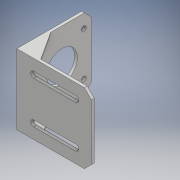
# Autodesk Inventor part: mount-extruder
Saved by Autodesk Inventor 2018 (Build 220112000, 112)
## iProperties
Created: 2017-10-21
Part Number: mount-extruder
Material: Generic
Document SubType Name: Modeling
Designer: Jurjen
Density: 1 g/cm^3
Appearance: Default
Author: Jurjen
Autodesk Inventor part; units mm, degrees
ref_plane "YZ Plane" through (0, 0, 0) normal (1, 0, 0) x (0, 1, 0)
ref_plane "XZ Plane" through (0, 0, 0) normal (0, 1, 0) x (-1, 0, 0)
ref_plane "XY Plane" through (0, 0, 0) normal (0, 0, 1) x (1, 0, 0)
sketch "Sketch1" plane through (0, 0, 0) normal (0, 0, 1) x (1, 0, 0)
  line L0 (-26.5, 25.5) -> (-24.5, 25.5)
  line L1 (-24.5, 25.5) -> (-24.5, -23.5)
  line L2 (-26.5, -25.5) -> (26.5, -25.5)
  line L3 (26.5, -25.5) -> (26.5, -23.5)
  line L4 (26.5, -23.5) -> (-24.5, -23.5)
  line L5 (-26.5, 25.5) -> (-26.5, -25.5)
  point P0 (0, 0)
  point P1 (-26.5, 0)
  point P2 (0, -25.5)
  dimension "d1" = 51
  dimension "d2" = 2
  dimension "d4" = 2
  dimension "d5" = 53
  constraints: 12 end point, 2 horizontal, 2 midpoint, 2 parallel, 2 perpendicular, 1 horizontal alignment, 1 vertical alignment
  measures "d1" distance of L0.start L2.start
  measures "d2" distance between parallel lines of L2 L4
  measures "d4" distance between parallel lines of L1 L5
  measures "d5" distance between parallel lines of L3 L5
extrude "Extrusion1" add sketch "Sketch1" along normal mid plane 50
sketch "Sketch2" plane through (-24.5, -23.5, 25) normal (1, 0, 0) x (0, 0, -1)
  circle A0 centre (25, 28) radius 11.05
  circle A1 centre (9.5, 43.5) radius 1.75
  circle A2 centre (40.5, 43.5) radius 1.75
  circle A3 centre (9.5, 12.5) radius 1.75
  circle A4 centre (40.5, 12.5) radius 1.75
  line L0 (0, 49) -> (50, 49) projected
  line L1 (9.5, 43.5) -> (40.5, 43.5) construction
  line L2 (9.5, 43.5) -> (9.5, 12.5) construction
  point P0 (25, 23.5)
  point P1 (25, 43.5)
  point P2 (9.5, 28)
  dimension "d8" = 22.1
  dimension "d9" = 3.5
  dimension "d10" = 31
  dimension "d11" = 31
  dimension "d12" = 21
  constraints: 5 centre point, 4 end point, 4 vertical alignment, 3 equal radius, 3 horizontal alignment, 2 midpoint, 1 horizontal, 1 vertical
  measures "d8" diameter of A0
  measures "d9" diameter of A1
  measures "d10" distance of L1.end L1.start
  measures "d11" distance of A4.centre L1.end
  measures "d12" distance from line of A0.centre L0
extrude "Extrusion2" cut sketch "Sketch2" against normal up to next
sketch "Sketch3" plane through (-24.5, -23.5, 25) normal (1, 0, 0) x (0, 0, -1)
  line L0 (0, 44) -> (5, 49)
  line L1 (50, 49) -> (0, 49) projected
  line L2 (25, 22.7162) -> (25, 49) construction
  line L3 (50, 44) -> (45, 49)
  line L4 (0, 0) -> (0, 49) projected
  line L5 (50, 49) -> (50, 0) projected
  line L6 (0, 49) -> (50, 49) projected
  line L7 (45, 49) -> (50, 49)
  line L8 (50, 49) -> (50, 44)
  line L9 (5, 49) -> (0, 49)
  line L10 (0, 44) -> (0, 49)
  point P0 (25, 23.5)
  dimension "d15" = 45
  dimension "d16" = 5
  constraints: 14 end point, 3 collinear, 2 symmetric about line, 2 vertical alignment, 1 midpoint, 1 perpendicular, 1 point on line
  measures "d15" angle of L1 L0
  measures "d16" distance of L1.end L0.end
extrude "Extrusion3" cut sketch "Sketch3" against normal up to next
sketch "Sketch4" plane through (-24.5, -23.5, 25) normal (0, 1, 0) x (1, 0, 0)
  arc A0 (10, 12.1) -> (10, 7.9) centre (10, 10) ccw
  arc A1 (10, 42.1) -> (10, 37.9) centre (10, 40) ccw
  arc A2 (40, 7.9) -> (40, 12.1) centre (40, 10) ccw
  arc A3 (40, 37.9) -> (40, 42.1) centre (40, 40) ccw
  line L0 (40, 7.9) -> (10, 7.9)
  line L1 (10, 12.1) -> (40, 12.1)
  line L2 (10, 37.9) -> (40, 37.9)
  line L3 (10, 42.1) -> (40, 42.1)
  line L4 (10, 10) -> (10, 40) construction
  line L5 (51, 50) -> (51, 0) projected
  point P0 (24.5, 25)
  point P1 (10, 25)
  dimension "d19" = 4.2
  dimension "d20" = 30
  dimension "d21" = 30
  dimension "d22" = 4.2
  dimension "d23" = 11
  constraints: 10 end point, 8 point on circle, 4 centre point, 3 equal radius, 3 horizontal alignment, 3 parallel, 3 tangent, 2 vertical alignment, 1 horizontal, 1 midpoint, 1 vertical
  measures "d19" diameter of A0
  measures "d20" distance of L4.start L4.end
  measures "d21" distance of L4.start A2.centre
  measures "d22" distance between parallel lines of L3 L2
  measures "d23" distance from line of L5 A3.centre
extrude "Extrusion4" cut sketch "Sketch4" against normal up to next
sketch "Sketch5" plane through (-24.5, -23.5, 25) normal (0, 1, 0) x (1, 0, 0)
  line L0 (10, 12.1) -> (40, 12.1) projected
  arc A0 (40, 7.9) -> (40, 12.1) centre (40, 10) ccw projected
  line L1 (40, 7.9) -> (10, 7.9) projected
  arc A1 (10, 12.1) -> (10, 7.9) centre (10, 10) ccw projected
  line L2 (40, 37.9) -> (10, 37.9) projected
  arc A2 (10, 42.1) -> (10, 37.9) centre (10, 40) ccw projected
  line L3 (10, 42.1) -> (40, 42.1) projected
  arc A3 (40, 37.9) -> (40, 42.1) centre (40, 40) ccw projected
  line L4 (0, 50) -> (0, 0) projected
  line L5 (51, 0) -> (0, 0) projected
  line L6 (51, 50) -> (51, 0) projected
  line L7 (0, 50) -> (51, 50) projected
  line L8 (46, 0) -> (51, 5)
  line L9 (51, 45) -> (46, 50)
  line L10 (51, 50) -> (-2, 50) projected
  point P0 (24.5, 25)
  dimension "d26" = 5
  dimension "d27" = 5
  constraints: 4 end point, 4 point on line, 2 vertical alignment, 1 perpendicular
  measures "d26" distance from line of L8.start L6
  measures "d27" distance of L5.start L8.end
extrude "Extrusion5" cut sketch "Sketch5" against normal up to next contours L7 L6 L9 | L8 L6 L5
sketch "Sketch6" plane through (0, 0, 25) normal (0, 0, 1) x (1, 0, 0)
  line L0 (-11.5, -23.5) -> (-24.5, -3.5)
  line L1 (-11.5, -23.5) -> (-24.5, -23.5)
  line L2 (-24.5, -23.5) -> (-24.5, -3.5)
  point P0 (0, 0)
  dimension "d30" = 13
  dimension "d31" = 20
  constraints: 6 end point, 1 horizontal, 1 horizontal alignment, 1 perpendicular, 1 vertical alignment
  measures "d30" distance of L0.start L1.end
  measures "d31" distance of L1.end L0.end
extrude "Extrusion6" add sketch "Sketch6" against normal blind 1
mirror "Mirror1" about plane through (0, 0, 0) normal (0, 0, 1) of "Extrusion6"
equation "\"d22\" = d19"
body "Solid1"
